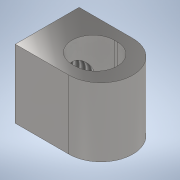
# Autodesk Inventor part: metal_connector
Saved by Autodesk Inventor 2021 (Build 250183000, 183)
## iProperties
Created: 2022-03-25
Part Number: metal_connector
Material: Steel, Alloy
Document SubType Name: Modeling
Designer: ermoz
Density: 7.73 g/cm^3
Appearance: Semi-Polished
Author: ermoz
Autodesk Inventor part; units mm, degrees
ref_plane "YZ Plane" through (0, 0, 0) normal (1, 0, 0) x (0, 1, 0)
ref_plane "XZ Plane" through (0, 0, 0) normal (0, 1, 0) x (-1, 0, 0)
ref_plane "XY Plane" through (0, 0, 0) normal (0, 0, 1) x (1, 0, 0)
sketch "Sketch1" plane through (0, 0, 0) normal (0, 1, 0) x (-1, 0, 0)
  circle A0 centre (-0.4, 0) radius 2.05
  line L0 (-0.4, 2.05) -> (3.05, 2.05)
  line L1 (3.05, 2.05) -> (3.05, -2.05)
  line L2 (3.05, -2.05) -> (-0.4, -2.05)
  line L3 (-2.45, 0) -> (-2.45, -1.163)
  line L4 (-1.45, 0) -> (1.45, 0) construction
  line L5 (-0.1, -1.35) -> (0.1, -1.35)
  line L6 (0.1, 1.35) -> (-0.1, 1.35)
  arc A1 (-0.1, 1.35) -> (-0.1, -1.35) centre (-0.1, 0) ccw
  arc A2 (0.1, -1.35) -> (0.1, 1.35) centre (0.1, 0) ccw
  point P0 (0, 0)
  point P1 (0, 0)
  dimension "d1" = 4.1
  dimension "d2" = 5.5
  dimension "d3" = 2.7
  dimension "d4" = 2.9
  dimension "d5" = 1
  constraints: 16 end point, 11 point on circle, 7 tangent, 3 centre point, 3 horizontal, 2 horizontal alignment, 2 point on line, 1 coincident, 1 midpoint, 1 parallel, 1 perpendicular, 1 vertical
  measures "d1" diameter of A0
  measures "d2" distance between parallel lines of L1 L3
  measures "d3" diameter of A2
  measures "d4" distance of L4.end L4.start
  measures "d5" distance of L3.start L4.start
extrude "Extrusion1" add sketch "Sketch1" along normal blind 4.4
sketch "Sketch2" plane through (-3.05, 0, -2.05) normal (-1, 0, 0) x (0, 0, 1)
  line L0 (0, 0) -> (4.1, 0) projected
  line L1 (4.1, 0) -> (4.1, 4.4) projected
  line L2 (0, 4.4) -> (4.1, 4.4) projected
  line L3 (0, 0) -> (0, 4.4) projected
  circle A0 centre (2.05, 2.2) radius 1
  point P0 (2.05, 0)
  dimension "d8" = 2
  constraints: 1 centre point
  measures "d8" diameter of A0
extrude "Extrusion2" cut sketch "Sketch2" against normal up to surface contours A0
thread "Thread1" size "M2x0.4" class "6H" standard "ANSI Metric M Profile" full length
chamfer "Chamfer1" distance 0.2 angle 45 1 edges at (-3.05, 2.2, -1)
body "Solid1"
